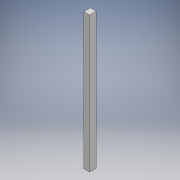
# Autodesk Inventor part: PL_rod_single
Saved by Autodesk Inventor 2018.3 (Build 223284000, 284)
## iProperties
Created: 2020-08-29
Part Number: PL_rod_single
Material: Generic
Document SubType Name: Modeling
Designer: chris
Density: 1 g/cm^3
Appearance: Default
Author: chris
Autodesk Inventor part; units mm, degrees
ref_plane "YZ Plane" through (0, 0, 0) normal (1, 0, 0) x (0, 1, 0)
ref_plane "XZ Plane" through (0, 0, 0) normal (0, 1, 0) x (-1, 0, 0)
ref_plane "XY Plane" through (0, 0, 0) normal (0, 0, 1) x (1, 0, 0)
sketch "Sketch1" plane through (0, 0, 0) normal (0, 0, 1) x (1, 0, 0)
  line L0 (-7.2, -8.1) -> (7.2, -8.1)
  line L1 (7.2, -8.1) -> (7.2, 8.1)
  line L2 (7.2, 8.1) -> (-7.2, 8.1)
  line L3 (-7.2, 8.1) -> (-7.2, -8.1)
  line L4 (-6.2, 7.1) -> (6.2, 7.1)
  line L5 (6.2, 7.1) -> (6.2, -7.1)
  line L6 (6.2, -7.1) -> (-6.2, -7.1)
  line L7 (-6.2, -7.1) -> (-6.2, 7.1)
  dimension "d9" = 1
  constraints: 16 end point, 4 parallel, 2 perpendicular, 1 horizontal, 3 other
  measures "d9" distance between parallel lines of L2 L4
extrude "Extrusion2" add sketch "Sketch1" along normal blind 340
sketch "Sketch2" plane through (0, 0, 340) normal (0, 0, 1) x (1, 0, 0)
  line L0 (-7.2, -8.1) -> (7.2, -8.1) construction
  line L1 (-7.2, 8.1) -> (7.2, 8.1)
  line L2 (7.2, 8.1) -> (7.2, -8.1)
  line L3 (7.2, -8.1) -> (-7.2, -8.1)
  line L4 (-7.2, -8.1) -> (-7.2, 8.1)
  point P0 (0, 0)
  constraints: 8 end point, 2 parallel, 1 horizontal, 1 perpendicular
extrude "Extrusion3" add sketch "Sketch2" against normal blind 2
sketch "Sketch3" plane through (0, 0, 0) normal (0, 0, -1) x (-1, 0, 0)
  line L0 (-7.2, -8.1) -> (-7.2, 8.1) construction
  line L1 (7.2, 8.1) -> (7.2, -8.1) construction
  line L2 (-7.2, -8.1) -> (7.2, -8.1)
  line L3 (7.2, -8.1) -> (7.2, 8.1)
  line L4 (7.2, 8.1) -> (-7.2, 8.1)
  line L5 (-7.2, 8.1) -> (-7.2, -8.1)
  point P0 (0, 0)
  constraints: 8 end point, 2 parallel, 1 horizontal, 1 perpendicular
extrude "Extrusion4" add sketch "Sketch3" against normal blind 2
body "Solid2"
